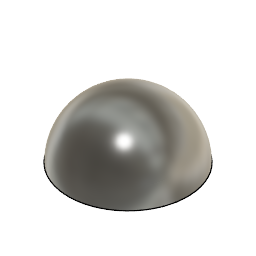
BOQUILLA (Autodesk Fusion 360 design; units mm, degrees)
Autodesk Fusion 360 part; units mm, degrees
sketch "Sketch1" plane through (0, 0, 0) normal (0, 0, 1) x (1, 0, 0)
  circle A0 centre (0, 0) radius 17.5
  line L0 (-45.9409, 0) -> (53.3167, 0)
  dimension "d1" = 35
  constraint coincident A0.centre origin
  constraint horizontal L0
  constraint coincident A0.centre L0
  measures "d1" diameter of A0
revolve "Revolve1" add sketch "Sketch1" angle 180 about axis through (-45.9409, 0, 0) along (1, 0, 0) contours A0 L0 picked at (-3.4943, 10.2478)
shell "Shell1" thickness 2 removed faces 2 at (-3.4943, 10.2478, 0) at (-3.4943, -10.2478, 0)
